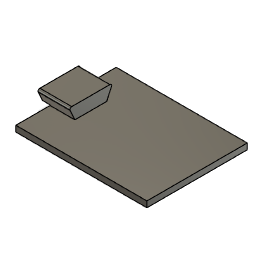
charger (Autodesk Fusion 360 design; units mm, degrees)
Autodesk Fusion 360 part; units mm, degrees
sketch "Sketch1" plane through (0, 0, 0) normal (0, 1, 0) x (1, 0, 0)
  line L0 (0, 0) -> (22.2, 0)
  line L1 (22.2, 0) -> (22.2, 17)
  line L2 (22.2, 17) -> (0, 17)
  line L3 (0, 17) -> (0, 0)
  dimension "d1" = 22.2
  dimension "d2" = 17
  constraint horizontal L0
  constraint vertical L1
  constraint horizontal L2
  constraint vertical L3
  constraint coincident L0.start L3.end
  measures "d1" distance of L0.start L0.end
  measures "d2" distance of L0.start L2.end
extrude "Extrude1" add sketch "Sketch1" along normal blind 1
sketch "Sketch2" plane through (0, 0, 0) normal (-1, 0, 0) x (0, 0, 1)
  line L0 (-17, 0) -> (0, 0)
  line L1 (0, 0) -> (0, 1)
  line L2 (0, 1) -> (-17, 1)
  line L3 (-17, 1) -> (-17, 0)
  line L4 (-12.2, 3.2) -> (-4.8, 3.2)
  line L5 (-4.8, 3.2) -> (-5.7974, 1)
  line L6 (-11.1974, 1) -> (-12.2, 3.2)
  point P0 (-8.5, 1)
  point P1 (-8.5, 3.2)
  dimension "d5" = 7.4
  dimension "d6" = 5.4
  dimension "d7" = 2.2
  dimension "d8" = 114.5
  constraint horizontal L4
  constraint coincident L2 L5.end
  constraint coincident L2 L6.start
  constraint midpoint L2 P0
  constraint midpoint L4 P1
  constraint vertical P0 P1
  measures "d5" distance of L4.start L4.end
  measures "d6" distance of L5.end L6.start
  measures "d7" distance of L4 L5.end
  measures "d8" angle of L2 L6
extrude "Extrude2" add sketch "Sketch2" along normal blind 1.2 and the other way blind 4.2 contours L2 L4 L5 L6
fillet "Fillet1" radius 0.3 4 edges at (1.5, 3.2, -4.8) (1.5, 3.2, -12.2) (-0.6, 1, -5.7974) (-0.6, 1, -11.1974)
